Autodesk Fusion 360 part; units mm, degrees
note: some values were not read from the file. Chosen so that the rebuilt part matches the saved one: which face or edge a step refers to. Set by a fixed rule: which sketch regions a step uses.
(part 3 of 4)
sketch "Contents" plane through (0, 0, 0) normal (0, 0, 1) x (1, 0, 0) in component "Brace"
  circle A0 centre (34, 34.6) radius 15
  line L0 (40, 122) -> (22, 122)
  line L1 (60, 0) -> (0, 0) construction
  line L2 (18.5, 19.1) -> (18.5, 50.1) construction
  circle A1 centre (53, 31) radius 1.25
  circle A2 centre (53, 61) radius 1.25
  circle A3 centre (53, 121) radius 1.25
  line L3 (0, 0) -> (0, 182) construction
  line L4 (49.5, 19.1) -> (18.5, 50.1) construction
  circle A4 centre (18.5, 50.1) radius 1.5
  circle A5 centre (53, 91) radius 1.25
  line L5 (49.5, 50.1) -> (49.5, 19.1) construction
  line L6 (22, 162) -> (40, 162)
  line L7 (18.5, 19.1) -> (49.5, 50.1) construction
  circle A6 centre (53, 151) radius 1.25
  circle A7 centre (49.5, 19.1) radius 1.5
  line L8 (18.5, 50.1) -> (49.5, 50.1) construction
  line L9 (49.5, 19.1) -> (18.5, 19.1) construction
  line L10 (0, 182) -> (60, 182) construction
  circle A8 centre (18.5, 19.1) radius 1.5
  circle A9 centre (49.5, 50.1) radius 1.5
  line L11 (40, 162) -> (40, 122)
  line L12 (60, 182) -> (60, 0) construction
  line L13 (3.175, 95) -> (13.175, 95)
  line L14 (13.175, 95) -> (13.175, 87)
  line L15 (13.175, 87) -> (3.175, 87)
  line L16 (0, 425.6) -> (0, -184)
  line L17 (27.6442, 147.907) -> (28.3894, 146.7583)
  line L18 (34.519, 148.0232) -> (33.9924, 147.4295)
  arc A10 (33.9924, 147.4295) -> (27.6442, 147.907) centre (31, 150.0839) ccw
  line L19 (32, 141.3873) -> (32, 132.9489)
  line L20 (30, 132.9489) -> (30, 141.316)
  line L21 (31.1201, 154.0821) -> (30.7651, 146.624) construction
  line L22 (30, 132.9489) -> (32, 132.9489)
  arc A11 (34.519, 148.0232) -> (32, 141.3873) centre (42, 141.3873) ccw
  arc A12 (30, 141.316) -> (28.3894, 146.7583) centre (20, 141.316) ccw
  line L23 (31, 150.0839) -> (31, 109.1329) construction
  line L24 (19.1457, 161.9685) -> (15.5387, 161.9685)
  line L25 (15.5387, 161.9685) -> (15.5387, 153.7089)
  line L26 (19.1457, 161.1035) -> (22, 161.1035)
  line L27 (22, 158.4561) -> (22, 154.2014)
  line L28 (19.1457, 157.1289) -> (19.1457, 158.4561)
  line L29 (19.1457, 158.4561) -> (22, 158.4561)
  line L30 (22, 158.4561) -> (22, 157.1289)
  line L31 (19.1457, 153.7089) -> (19.1457, 158.4561)
  line L32 (19.1457, 161.1035) -> (19.1457, 161.9685)
  line L33 (15.5387, 153.7089) -> (19.1457, 153.7089)
  line L34 (22, 122) -> (22, 158.4561)
  line L35 (22, 161.1035) -> (22, 162)
  point P0 (60, 91)
  point P1 (34, 34.6)
  point P2 (0, 182)
  dimension "d1134" = 33
  dimension "d1135" = -30
  dimension "d1136" = 182
  dimension "d1137" = 60
  dimension "d974" = 2.5
  dimension "d975" = 7
  dimension "d1140" = 31
  dimension "d1141" = 31
  dimension "d1142" = 30
  dimension "d1143" = 3
  dimension "d1144" = 3
  dimension "d1145" = 3
  dimension "d1146" = 3
  dimension "d1147" = 26
  dimension "d1148" = 34.6
  dimension "d1149" = 20
  dimension "d1011" = 20
  dimension "d1012" = 18
  dimension "d1013" = 40
  dimension "d1716" = 3.175
  dimension "d1717" = 8
  dimension "d1718" = 87
  dimension "d1719" = 10
  dimension "d1720" = 9
  dimension "d1721" = 8
  dimension "d1722" = 2
  dimension "d1723" = 10
  dimension "d1724" = 10
  constraint perpendicular L1 L12
  constraint parallel L3 L12
  constraint coincident P2 L3.end
  constraint perpendicular L10 L12
  constraint midpoint P0 L12
  constraint horizontal P0 A5.centre
  constraint horizontal L9
  constraint perpendicular L2 L9
  constraint parallel L8 L9
  constraint parallel L2 L5
  constraint coincident P1 L4
  constraint coincident P1 L7
  constraint coincident P1 A0.centre
  constraint coincident L2.end L4.end
  constraint coincident L5.start L7.end
  constraint coincident L4.start L5.end
  constraint coincident L2.start L7.start
  constraint horizontal L6
  constraint vertical L11
  constraint horizontal L0
  constraint vertical L34
  constraint coincident L1.end L3.start
  constraint horizontal L13
  constraint vertical L14
  constraint horizontal L15
  constraint tangent L18 A10
  constraint tangent L17 A10
  constraint parallel L19 L20
  constraint coincident A10 L21.start
  constraint horizontal L22
  constraint tangent L18 A11
  constraint tangent L19 A11
  constraint tangent L17 A12
  constraint tangent L20 A12
  constraint coincident A10.centre L23.start
  constraint perpendicular L0 L23
  constraint horizontal L24
  constraint vertical L25
  constraint vertical L31
  constraint horizontal L26
  constraint vertical L27
  constraint coincident L27.end L34
  constraint coincident L26.start L31
  constraint vertical L28
  constraint horizontal L29
  constraint vertical L30
  constraint coincident L30.end L34
  constraint collinear L31 L32
  constraint perpendicular L31 L33
  constraint coincident L26.end L34
  constraint collinear L34 L35
  measures "d1136" distance of L1.end P2
  measures "d1137" distance of L1.end L1.start
  measures "d974" diameter of A5
  measures "d975" distance of A5.centre L12
  measures "d1140" distance of L2.end L5.start
  measures "d1141" distance of L2.end L2.start
  measures "d1142" diameter of A0
  measures "d1143" diameter of A4
  measures "d1144" diameter of A9
  measures "d1145" diameter of A7
  measures "d1146" diameter of A8
  measures "d1147" distance of P1 L12
  measures "d1148" distance of P1 L1
  measures "d1149" distance of L6.start L10
  measures "d1011" distance of L11 L12
  measures "d1012" distance of L0.end L0.start
  measures "d1013" distance of L0.end L6.start
  measures "d1716" distance of L13.start L16
  measures "d1717" distance of L13.end L14.end
  measures "d1718" distance of L10 L13
  measures "d1719" distance of L13.start L13.end
  measures "d1720" distance of A10.centre L34
  measures "d1721" diameter of A10
  measures "d1722" distance of L19.end L20.start
  measures "d1723" radius of A11
  measures "d1724" radius of A12
sketch "Content" plane through (0, 0, 0) normal (0, 0, 1) x (1, 0, 0) in component "Top"
  line L0 (-132, 172) -> (-116, 172)
  circle A0 centre (-49, 80) radius 1.5
  circle A1 centre (-49, 102) radius 1.5
  line L1 (0, 0) -> (-240, 0) construction
  line L2 (-114, 170) -> (-114, 127.9999)
  line L3 (-240, 182) -> (0, 182) construction
  line L4 (0, 182) -> (0, 0) construction
  circle A2 centre (-58, 151) radius 1.5
  circle A3 centre (-53, 136) radius 1.5
  circle A4 centre (-48, 151) radius 1.5
  circle A5 centre (-68, 146) radius 1.5
  circle A6 centre (-48, 146) radius 1.5
  circle A7 centre (-48, 156) radius 1.5
  circle A8 centre (-58, 156) radius 1.5
  circle A9 centre (-63, 141) radius 1.5
  circle A10 centre (-63, 151) radius 1.5
  circle A11 centre (-63, 146) radius 1.5
  circle A12 centre (-48, 141) radius 1.5
  circle A13 centre (-58, 146) radius 1.5
  circle A14 centre (-68, 151) radius 1.5
  line L5 (-163.976, 90) -> (-163.976, 96)
  circle A15 centre (-68, 136) radius 1.5
  circle A16 centre (-63, 156) radius 1.5
  circle A17 centre (-68, 156) radius 1.5
  circle A18 centre (-48, 136) radius 1.5
  circle A19 centre (-58, 136) radius 1.5
  line L6 (-240, 0) -> (-240, 182) construction
  circle A20 centre (-191, 102) radius 1.5
  circle A21 centre (-53, 156) radius 1.5
  circle A22 centre (-191, 80) radius 1.5
  line L7 (-134, 128) -> (-134, 170)
  circle A23 centre (-53, 146) radius 1.5
  line L8 (-159.976, 88) -> (-161.976, 88)
  line L9 (-161.976, 98) -> (-159.976, 98)
  circle A24 centre (-63, 136) radius 1.5
  line L10 (-157.976, 96) -> (-157.976, 90)
  circle A25 centre (-53, 141) radius 1.5
  circle A26 centre (-58, 141) radius 1.5
  circle A27 centre (-53, 151) radius 1.5
  line L11 (-116, 125.9999) -> (-132, 126)
  circle A28 centre (-68, 141) radius 1.5
  line L12 (0, 1.75) -> (0, 22.5)
  line L13 (1.75, 0) -> (22.5, 0)
  circle A29 centre (-68, 131) radius 1.5
  circle A30 centre (-63, 131) radius 1.5
  circle A31 centre (-58, 131) radius 1.5
  circle A32 centre (-53, 131) radius 1.5
  circle A33 centre (-48, 131) radius 1.5
  arc A34 (-161.976, 98) -> (-163.976, 96) centre (-161.976, 96) ccw
  arc A35 (-163.976, 90) -> (-161.976, 88) centre (-161.976, 90) ccw
  arc A36 (-159.976, 88) -> (-157.976, 90) centre (-159.976, 90) ccw
  arc A37 (-157.976, 96) -> (-159.976, 98) centre (-159.976, 96) ccw
  arc A38 (-132, 172) -> (-134, 170) centre (-132, 170) ccw
  arc A39 (-114, 170) -> (-116, 172) centre (-116, 170) ccw
  arc A40 (-116, 125.9999) -> (-114, 127.9999) centre (-116, 127.9999) ccw
  arc A41 (-134, 128) -> (-132, 126) centre (-132, 128) ccw
  line L14 (-131.3, 149.5) -> (-115.3, 149.5)
  circle A42 centre (-47, 47) radius 1.5
  circle A43 centre (-37, 62) radius 1.5
  circle A44 centre (-52, 47) radius 1.5
  circle A45 centre (-57, 67) radius 1.5
  circle A46 centre (-57, 57) radius 1.5
  circle A47 centre (-47, 67) radius 1.5
  circle A48 centre (-52, 57) radius 1.5
  circle A49 centre (-57, 47) radius 1.5
  circle A50 centre (-42, 62) radius 1.5
  circle A51 centre (-52, 52) radius 1.5
  circle A52 centre (-47, 62) radius 1.5
  circle A53 centre (-37, 52) radius 1.5
  circle A54 centre (-47, 52) radius 1.5
  circle A55 centre (-57, 62) radius 1.5
  circle A56 centre (-47, 57) radius 1.5
  circle A57 centre (-52, 67) radius 1.5
  circle A58 centre (-42, 52) radius 1.5
  circle A59 centre (-42, 57) radius 1.5
  circle A60 centre (-57, 52) radius 1.5
  circle A61 centre (-42, 47) radius 1.5
  circle A62 centre (-37, 67) radius 1.5
  circle A63 centre (-52, 62) radius 1.5
  circle A64 centre (-42, 67) radius 1.5
  circle A65 centre (-37, 57) radius 1.5
  circle A66 centre (-37, 47) radius 1.5
  line L15 (-242, 182) -> (-242, 0)
  circle A67 centre (-57, 42) radius 1.5
  circle A68 centre (-52, 42) radius 1.5
  circle A69 centre (-47, 42) radius 1.5
  circle A70 centre (-42, 42) radius 1.5
  circle A71 centre (-37, 42) radius 1.5
  circle A72 centre (-210, 15) radius 1.5
  circle A73 centre (-215, 30) radius 1.5
  circle A74 centre (-205, 25) radius 1.5
  circle A75 centre (-205, 30) radius 1.5
  circle A76 centre (-195, 20) radius 1.5
  circle A77 centre (-200, 30) radius 1.5
  circle A78 centre (-210, 20) radius 1.5
  circle A79 centre (-205, 15) radius 1.5
  circle A80 centre (-210, 30) radius 1.5
  circle A81 centre (-210, 10) radius 1.5
  circle A82 centre (-200, 10) radius 1.5
  circle A83 centre (-210, 25) radius 1.5
  circle A84 centre (-215, 25) radius 1.5
  circle A85 centre (-215, 15) radius 1.5
  circle A86 centre (-200, 25) radius 1.5
  circle A87 centre (-200, 20) radius 1.5
  circle A88 centre (-215, 10) radius 1.5
  circle A89 centre (-215, 20) radius 1.5
  circle A90 centre (-205, 10) radius 1.5
  circle A91 centre (-195, 10) radius 1.5
  circle A92 centre (-195, 25) radius 1.5
  circle A93 centre (-205, 20) radius 1.5
  circle A94 centre (-195, 15) radius 1.5
  circle A95 centre (-195, 30) radius 1.5
  circle A96 centre (-200, 15) radius 1.5
  line L16 (-240, 0) -> (-240, 182)
  circle A97 centre (-128.0762, 158.5418) radius 1.6
  circle A98 centre (-128.0762, 158.5418) radius 3.5
  circle A99 centre (-119.0762, 158.5418) radius 1.6
  circle A100 centre (-119.0762, 158.5418) radius 3.5
  circle A101 centre (-128.0762, 167.5418) radius 1.6
  circle A102 centre (-128.0762, 167.5418) radius 3.5
  circle A103 centre (-119.0762, 167.5418) radius 1.6
  circle A104 centre (-119.0762, 167.5418) radius 3.5
  arc A105 (-124.6, 139.8073) -> (-127.2667, 146.606) centre (-134.6, 139.8073) ccw
  line L17 (-124.6, 128.3707) -> (-122.8, 152.6283) construction
  arc A106 (-119.9333, 146.606) -> (-122.6, 139.8073) centre (-112.6, 139.8073) ccw
  line L18 (-124.6, 128.3707) -> (-124.6, 139.8073)
  line L19 (-122.6, 128.3707) -> (-124.6, 128.3707)
  line L20 (-122.6, 128.3707) -> (-124.6, 152.6283) construction
  line L21 (-122.6, 139.8073) -> (-122.6, 128.3707)
  arc A107 (-119.9333, 146.606) -> (-127.2667, 146.606) centre (-123.6, 150.0053) ccw
  point P0 (-134, 172)
  point P1 (-160.976, 126.0001)
  point P2 (-157.976, 98)
  point P3 (-114, 172)
  point P4 (-134, 126)
  point P5 (-160.976, 98)
  point P6 (-163.976, 98)
  point P7 (-163.976, 88)
  point P8 (-123.6526, 141.1379)
  dimension "d1161" = 142
  dimension "d1163" = 240
  dimension "d1164" = 182
  dimension "d1165" = 20
  dimension "d1166" = 46
  dimension "d1167" = 6
  dimension "d1168" = 10
  dimension "d1169" = 10
  dimension "d1170" = 106
  dimension "d1171" = 84
  dimension "d1172" = 26
  dimension "d1173" = 3
  dimension "d1174" = 68
  dimension "d1175" = 3
  dimension "d1176" = 49
  dimension "d1177" = 80
  dimension "d1600" = 2
  dimension "d1601" = 2
  dimension "d1602" = 2
  dimension "d1603" = 2
  dimension "d1604" = 2
  dimension "d1605" = 2
  dimension "d1606" = 2
  dimension "d1607" = 2
  dimension "d1696" = 3
  dimension "d1699" = 47
  dimension "d1700" = 47
  dimension "d1705" = 3
  dimension "d1707" = 30
  dimension "d1708" = 20
  dimension "d1709" = 3.2
  dimension "d1710" = 7
  dimension "d1713" = 9
  dimension "d1714" = 9
  dimension "d1739" = 1.8
  dimension "d1740" = 10
  dimension "d1741" = 10
  dimension "d1742" = 10
  constraint horizontal L3
  constraint perpendicular L3 L4
  constraint horizontal L0
  constraint vertical L2
  constraint vertical L7
  constraint horizontal L9
  constraint vertical L10
  constraint horizontal L8
  constraint vertical L5
  constraint vertical P1 P5
  constraint perpendicular L1 L6
  constraint collinear L4 L12
  constraint collinear L1 L13
  constraint coincident P5 L9
  constraint coincident P6 L9
  constraint coincident P6 L5
  constraint tangent L9 A34
  constraint tangent L5 A34
  constraint coincident P7 L8
  constraint coincident P7 L5
  constraint tangent L8 A35
  constraint tangent L5 A35
  constraint tangent L8 A36
  constraint tangent L10 A36
  constraint coincident P2 L10
  constraint coincident P2 L9
  constraint tangent L10 A37
  constraint tangent L9 A37
  constraint coincident P0 L0
  constraint coincident P0 L7
  constraint tangent L0 A38
  constraint tangent L7 A38
  constraint coincident P3 L0
  constraint coincident P3 L2
  constraint tangent L0 A39
  constraint tangent L2 A39
  constraint coincident P1 L11
  constraint tangent L11 A40
  constraint tangent L2 A40
  constraint coincident P4 L7
  constraint coincident P4 L11
  constraint tangent L7 A41
  constraint tangent L11 A41
  constraint equal L0 L11
  constraint midpoint P5 L9
  constraint concentric A97 A98
  constraint horizontal L19
  constraint perpendicular L18 L19
  constraint parallel L18 L21
  constraint coincident P8 L20
  constraint coincident P8 L17
  constraint tangent A106 A107
  constraint tangent A106 L21
  constraint tangent A105 A107
  constraint tangent A105 L18
  measures "d1163" distance of L3.end L3.start
  measures "d1164" distance of L1.end L3.start
  measures "d1165" distance of P0 P3
  measures "d1166" distance of P0 P4
  measures "d1167" distance of P2 P6
  measures "d1168" distance of P6 P7
  measures "d1169" distance of L0 L3
  measures "d1170" distance of L6 L7
  measures "d1171" distance of L3 L9
  measures "d1172" distance of A17.centre L3
  measures "d1173" diameter of A17
  measures "d1174" distance of A17.centre L4
  measures "d1175" diameter of A20
  measures "d1176" distance of A20.centre L6
  measures "d1177" distance of A20.centre L3
  measures "d1600" radius of A34
  measures "d1601" radius of A35
  measures "d1602" radius of A36
  measures "d1603" radius of A37
  measures "d1604" radius of A38
  measures "d1605" radius of A39
  measures "d1606" radius of A40
  measures "d1607" radius of A41
  measures "d1696" diameter of A45
  measures "d1699" distance of L4 A47.centre
  measures "d1700" distance of L1 A49.centre
  measures "d1705" diameter of A73
  measures "d1707" distance of A80.centre L16
  measures "d1708" distance of L1 A93.centre
  measures "d1709" diameter of A97
  measures "d1710" diameter of A98
  measures "d1739" distance of L20.end L17.end
  measures "d1740" diameter of A107
  measures "d1741" radius of A106
  measures "d1742" radius of A105
sketch "Content (2)" plane through (0, 0, 0) normal (0, 0, 1) x (1, 0, 0) in component "Bottom"
  line L0 (-240, -184) -> (-240, -2) construction
  line L1 (-240, -2) -> (0, -2) construction
  line L2 (0, -184) -> (-240, -184) construction
  circle A0 centre (-139, -9) radius 1
  circle A1 centre (-15, -172) radius 1.75
  line L3 (0, -2) -> (0, -184) construction
  circle A2 centre (-120, -93.901) radius 1.05
  circle A3 centre (-225, -172) radius 1.75
  circle A4 centre (-225, -17) radius 1.75
  circle A5 centre (-139, -103) radius 1
  circle A6 centre (-15, -17) radius 1.75
  circle A7 centre (-233, -103) radius 1
  circle A8 centre (-233, -9) radius 1
  line L4 (1.75, 0) -> (22.5, 0) construction
  line L5 (0, 1.75) -> (0, 22.5) construction
  line L6 (0, -184) -> (-304.8, -184)
  circle A9 centre (-76.675, -120) radius 2
  circle A10 centre (-26.675, -120) radius 2
  circle A11 centre (-76.675, -151) radius 2
  circle A12 centre (-26.675, -151) radius 2
  line L7 (0, 425.6) -> (0, -184)
  circle A13 centre (-211.0542, -25.3538) radius 1.0005
  circle A14 centre (-157.9209, -25.3538) radius 1.0005
  circle A15 centre (-104.7876, -25.3538) radius 1.0005
  circle A16 centre (-51.6542, -25.3538) radius 1.0005
  circle A17 centre (-211.0542, -68.4205) radius 1.0005
  circle A18 centre (-157.9209, -68.4205) radius 1.0005
  circle A19 centre (-51.6542, -68.4205) radius 1.0005
  circle A20 centre (-211.0542, -111.4871) radius 1.0005
  circle A21 centre (-51.6542, -111.4871) radius 1.0005
  circle A22 centre (-211.0542, -154.5538) radius 1.0005
  circle A23 centre (-157.9209, -154.5538) radius 1.0005
  circle A24 centre (-104.7876, -154.5538) radius 1.0005
  circle A25 centre (-51.6542, -154.5538) radius 1.0005
  point P0 (-120, -93.901)
  point P1 (0, -2)
  dimension "d828" = 210
  dimension "d829" = -155
  dimension "d832" = 94
  dimension "d833" = -94
  dimension "d282" = 3.5
  dimension "d289" = 2
  dimension "d422" = 240
  dimension "d423" = 182
  dimension "d424" = 15
  dimension "d426" = 15
  dimension "d427" = 7
  dimension "d428" = 7
  dimension "d463" = 2.1
  dimension "d843" = 2
  dimension "d1634" = 4
  dimension "d1637" = 50
  dimension "d1638" = -31
  dimension "d1639" = 64
  dimension "d1640" = 26.675
  dimension "d1726" = 2.001
  dimension "d1729" = 159.4
  dimension "d1730" = -129.2
  constraint horizontal L2
  constraint perpendicular L0 L2
  constraint parallel L1 L2
  constraint coincident P0 A2.centre
  constraint coincident P1 L1.end
  constraint vertical L3
  constraint collinear L3 L5
  measures "d282" diameter of A4
  measures "d289" diameter of A8
  measures "d422" distance of P1 L0.end
  measures "d423" distance of L0.start L0.end
  measures "d424" distance of A4.centre L1
  measures "d426" distance of A4.centre L0
  measures "d427" distance of A8.centre L1
  measures "d428" distance of A8.centre L0
  measures "d463" diameter of A2
  measures "d843" distance of L1 L4
  measures "d1634" diameter of A9
  measures "d1639" distance of L2 A9.centre
  measures "d1640" distance of A12.centre L7
  measures "d1726" diameter of A13
sketch "Content (3)" plane through (0, 0, 0) normal (0, 0, 1) x (1, 0, 0) in component "Front"
  line L0 (242, 62) -> (2, 62) construction
  line L1 (2, 2) -> (242, 2) construction
  line L2 (2, 62) -> (2, 2) construction
  line L3 (242, 62) -> (242, 2) construction
  line L4 (0, 1.75) -> (0, 22.5) construction
  line L5 (1.75, 0) -> (22.5, 0) construction
  line L6 (39.175, 22.1755) -> (39.175, 46.6727) construction
  circle A0 centre (48.175, 16.175) radius 5
  circle A1 centre (48.175, 34.175) radius 9
  circle A2 centre (216.325, 32) radius 15
  circle A3 centre (216.325, 32) radius 1.5
  circle A4 centre (216.325, 56.5) radius 1.5
  circle A5 centre (216.325, 7.5) radius 1.5
  circle A6 centre (216.325, 32) radius 20.5 construction
  circle A7 centre (169.325, 32) radius 20.5 construction
  circle A8 centre (169.325, 32) radius 15
  circle A9 centre (169.325, 7.5) radius 1.5
  circle A10 centre (169.325, 32) radius 1.5
  circle A11 centre (169.325, 56.5) radius 1.5
  circle A12 centre (122.325, 32) radius 20.5 construction
  circle A13 centre (122.325, 32) radius 15
  circle A14 centre (122.325, 7.5) radius 1.5
  circle A15 centre (122.325, 32) radius 1.5
  circle A16 centre (122.325, 56.5) radius 1.5
  point P0 (1.401, 31.401)
  point P1 (47.095, 2)
  point P2 (242, 32)
  dimension "d492" = 240
  dimension "d493" = 60
  dimension "d1106" = 2
  dimension "d1400" = 2
  dimension "d1567" = 14.175
  dimension "d1568" = 10
  dimension "d1569" = 18
  dimension "d1570" = 18
  dimension "d1725" = 46.175
  dimension "d1746" = 30
  dimension "d1748" = 3
  dimension "d1751" = 0
  dimension "d1752" = -24.5
  dimension "d1753" = 41
  dimension "d1754" = 25.675
  dimension "d1757" = -47
  dimension "d1758" = 0
  constraint perpendicular L0 L2
  constraint perpendicular L0 L3
  constraint horizontal L1
  constraint vertical L6
  constraint vertical A0.centre A1.centre
  constraint tangent L6 A1
  constraint midpoint L3 P2
  constraint horizontal A2.centre P2
  constraint concentric A2 A3
  constraint concentric A2 A6
  measures "d492" distance of L0.end L0.start
  measures "d493" distance of L1.end L0.start
  measures "d1106" distance of L2 L4
  measures "d1400" distance of L1 L5
  measures "d1567" distance of L1 A0.centre
  measures "d1568" diameter of A0
  measures "d1569" diameter of A1
  measures "d1570" vertical distance of A0.centre A1.centre
  measures "d1725" distance of L2 A1.centre
  measures "d1746" diameter of A2
  measures "d1748" diameter of A3
  measures "d1753" diameter of A6
  measures "d1754" distance of L3 A2.centre
sketch "Content (4)" plane through (0, 0, 0) normal (0, 0, 1) x (1, 0, 0) in component "Back"
  line L0 (128, -33) -> (128, -39)
  line L1 (116, -39) -> (116, -33)
  circle A0 centre (172, -18) radius 1.75
  circle A1 centre (182, -28) radius 1.75
  circle A2 centre (182, -18) radius 1.75
  line L2 (2, -6) -> (2, -66) construction
  line L3 (119, -30) -> (125, -30)
  line L4 (242, -6) -> (2, -6) construction
  line L5 (2, -66) -> (242, -66) construction
  circle A3 centre (56, -27) radius 1.5
  circle A4 centre (172, -28) radius 1.75
  circle A5 centre (71, -17) radius 1.5
  circle A6 centre (56, -17) radius 1.5
  circle A7 centre (46, -32) radius 1.5
  circle A8 centre (223.2, -48) radius 5.5
  line L6 (242, -66) -> (242, -6) construction
  circle A9 centre (66, -32) radius 1.5
  circle A10 centre (66, -22) radius 1.5
  circle A11 centre (61, -32) radius 1.5
  circle A12 centre (41, -27) radius 1.5
  circle A13 centre (71, -32) radius 1.5
  circle A14 centre (46, -17) radius 1.5
  circle A15 centre (56, -22) radius 1.5
  circle A16 centre (66, -17) radius 1.5
  circle A17 centre (56, -32) radius 1.5
  circle A18 centre (66, -27) radius 1.5
  circle A19 centre (61, -22) radius 1.5
  circle A20 centre (61, -17) radius 1.5
  circle A21 centre (46, -22) radius 1.5
  circle A22 centre (51, -22) radius 1.5
  line L7 (125, -42) -> (119, -42)
  circle A23 centre (41, -32) radius 1.5
  circle A24 centre (51, -32) radius 1.5
  circle A25 centre (41, -17) radius 1.5
  circle A26 centre (71, -27) radius 1.5
  circle A27 centre (46, -27) radius 1.5
  circle A28 centre (51, -27) radius 1.5
  circle A29 centre (61, -27) radius 1.5
  circle A30 centre (51, -17) radius 1.5
  circle A31 centre (41, -22) radius 1.5
  circle A32 centre (71, -22) radius 1.5
  line L8 (0, 1.75) -> (0, 22.5) construction
  line L9 (1.75, 0) -> (22.5, 0) construction
  circle A33 centre (192, -18) radius 1.75
  circle A34 centre (202, -18) radius 1.75
  circle A35 centre (192, -28) radius 1.75
  circle A36 centre (202, -28) radius 1.75
  line L10 (14.1495, -52.3784) -> (48.441, -52.3784) construction
  line L11 (48.441, -52.3784) -> (48.441, -46.5889) construction
  line L12 (48.441, -46.5889) -> (14.1495, -46.5889) construction
  line L13 (14.1495, -46.5889) -> (14.1495, -52.3784) construction
  arc A37 (119, -30) -> (116, -33) centre (119, -33) ccw
  arc A38 (128, -33) -> (125, -30) centre (125, -33) ccw
  arc A39 (125, -42) -> (128, -39) centre (125, -39) ccw
  arc A40 (116, -39) -> (119, -42) centre (119, -39) ccw
  line L14 (227, -16) -> (227, -26)
  line L15 (220.6, -14) -> (225, -14)
  line L16 (225, -28) -> (220.6, -28)
  line L17 (218.6, -26) -> (218.6, -16)
  arc A41 (220.6, -14) -> (218.6, -16) centre (220.6, -16) ccw
  arc A42 (227, -16) -> (225, -14) centre (225, -16) ccw
  arc A43 (218.6, -26) -> (220.6, -28) centre (220.6, -26) ccw
  arc A44 (225, -28) -> (227, -26) centre (225, -26) ccw
  point P0 (242, -36)
  point P1 (116, -42)
  point P2 (116, -30)
  point P3 (128, -30)
  point P4 (218.6, -28)
  point P5 (218.6, -14)
  point P6 (227, -14)
  point P7 (223.2, -28)
  dimension "d1005" = 5
  dimension "d1006" = 5
  dimension "d1009" = 10
  dimension "d1010" = -10
  dimension "d502" = 240
  dimension "d503" = 60
  dimension "d696" = 18
  dimension "d866" = 12
  dimension "d867" = 12
  dimension "d869" = 24
  dimension "d870" = 3
  dimension "d1039" = 34
  dimension "d1041" = 12
  dimension "d1179" = 18.8
  dimension "d1180" = 114
  dimension "d1183" = 39
  dimension "d1047" = 2
  dimension "d1048" = 6
  dimension "d1561" = 3.5
  dimension "d1562" = 11
  dimension "d1563" = 70
  dimension "d1596" = 3
  dimension "d1597" = 3
  dimension "d1598" = 3
  dimension "d1599" = 3
  dimension "d1646" = 8.4
  dimension "d1647" = 14
  dimension "d1648" = 8
  dimension "d1654" = 2
  dimension "d1655" = 2
  dimension "d1656" = 2
  dimension "d1657" = 2
  dimension "d1658" = 15
  constraint horizontal L5
  constraint vertical L6
  constraint vertical L2
  constraint midpoint P0 L6
  constraint horizontal L4
  constraint horizontal L3
  constraint vertical L0
  constraint horizontal L7
  constraint vertical L1
  constraint coincident P2 L1
  constraint coincident P2 L3
  constraint tangent L1 A37
  constraint tangent L3 A37
  constraint coincident P3 L3
  constraint coincident P3 L0
  constraint tangent L3 A38
  constraint tangent L0 A38
  constraint tangent L0 A39
  constraint tangent L7 A39
  constraint coincident P1 L1
  constraint coincident P1 L7
  constraint tangent L1 A40
  constraint tangent L7 A40
  constraint horizontal L15
  constraint vertical L14
  constraint horizontal L16
  constraint vertical L17
  constraint vertical A8.centre P7
  constraint coincident P5 L17
  constraint coincident P5 L15
  constraint tangent L17 A41
  constraint tangent L15 A41
  constraint coincident P6 L15
  constraint coincident P6 L14
  constraint tangent L15 A42
  constraint tangent L14 A42
  constraint coincident L16 P7
  constraint coincident P4 L17
  constraint coincident P4 L16
  constraint tangent L17 A43
  constraint tangent L16 A43
  constraint tangent L14 A44
  constraint tangent L16 A44
  measures "d502" distance of L5.end L2.end
  measures "d503" distance of L2.end L2.start
  measures "d696" distance of A8.centre L5
  measures "d866" distance of P2 P3
  measures "d867" distance of P1 P2
  measures "d869" distance of L5 L7
  measures "d870" diameter of A23
  measures "d1039" distance of A23.centre L5
  measures "d1041" distance of A0.centre L4
  measures "d1179" distance of A8.centre L6
  measures "d1180" distance of L0 L6
  measures "d1183" distance of A23.centre L2
  measures "d1047" distance of L2 L8
  measures "d1048" distance of L4 L9
  measures "d1561" diameter of A0
  measures "d1562" diameter of A8
  measures "d1563" distance of A0.centre L6
  measures "d1596" radius of A37
  measures "d1597" radius of A38
  measures "d1598" radius of A39
  measures "d1599" radius of A40
  measures "d1646" distance of P5 P6
  measures "d1647" distance of P4 P5
  measures "d1648" distance of L4 L15
  measures "d1654" radius of A41
  measures "d1655" radius of A42
  measures "d1656" radius of A43
  measures "d1657" radius of A44
  measures "d1658" distance of L6 L14
sketch "Content (5)" plane through (0, 0, 0) normal (0, 0, 1) x (1, 0, 0) in component "Right"
  line L0 (-302, 182) -> (-242, 182) construction
  circle A0 centre (-275, 112) radius 5.75
  circle A1 centre (-277, 80) radius 1.75
  circle A2 centre (-287, 100) radius 1.75
  circle A3 centre (-277, 90) radius 1.75
  line L1 (-264.7, 57.5) -> (-267, 57.5)
  line L2 (-267, 45) -> (-264.7, 45)
  circle A4 centre (-287, 90) radius 1.75
  circle A5 centre (-287, 80) radius 1.75
  line L3 (-269, 55.5) -> (-269, 47)
  line L4 (-262.7, 47) -> (-262.7, 55.5)
  circle A6 centre (-297, 151) radius 1
  circle A7 centre (-277, 100) radius 1.75
  circle A8 centre (-297, 61) radius 1
  circle A9 centre (-297, 121) radius 1
  circle A10 centre (-297, 91) radius 1
  line L5 (-242, 182) -> (-242, 0) construction
  circle A11 centre (-297, 31) radius 1
  line L6 (-302, 0) -> (-302, 182) construction
  circle A12 centre (-267, 80) radius 1.75
  line L7 (-242, 0) -> (-302, 0) construction
  circle A13 centre (-267, 90) radius 1.75
  circle A14 centre (-267, 100) radius 1.75
  line L8 (1.75, 0) -> (22.5, 0) construction
  line L9 (0, 1.75) -> (0, 22.5) construction
  arc A15 (-262.7, 55.5) -> (-264.7, 57.5) centre (-264.7, 55.5) ccw
  arc A16 (-267, 57.5) -> (-269, 55.5) centre (-267, 55.5) ccw
  arc A17 (-269, 47) -> (-267, 45) centre (-267, 47) ccw
  arc A18 (-264.7, 45) -> (-262.7, 47) centre (-264.7, 47) ccw
  point P0 (-242, 91)
  point P1 (-262.7, 45)
  point P2 (-272, 0)
  point P3 (-269, 45)
  point P4 (-269, 57.5)
  point P5 (-302, 182)
  point P6 (-272, 182)
  dimension "d960" = -10
  dimension "d961" = -10
  dimension "d964" = 0
  dimension "d965" = -30
  dimension "d846" = 2
  dimension "d910" = 182
  dimension "d911" = 60
  dimension "d923" = 11.5
  dimension "d924" = 70
  dimension "d925" = 27
  dimension "d927" = 33
  dimension "d929" = 6.3
  dimension "d930" = 3.5
  dimension "d1192" = 100
  dimension "d1194" = 91
  dimension "d992" = 12.5
  dimension "d993" = 242
  dimension "d1538" = 45
  dimension "d1540" = 15
  dimension "d1564" = 5
  dimension "d1642" = 2
  dimension "d1643" = 2
  dimension "d1644" = 2
  dimension "d1645" = 2
  constraint perpendicular L5 L7
  constraint parallel L5 L6
  constraint coincident P5 L0.start
  constraint perpendicular L0 L5
  constraint midpoint P2 L7
  constraint midpoint P6 L0
  constraint horizontal L2
  constraint horizontal L1
  constraint vertical L3
  constraint midpoint P0 L5
  constraint perpendicular L1 L4
  constraint collinear L7 L8
  constraint tangent L1 A15
  constraint tangent L4 A15
  constraint coincident P4 L1
  constraint coincident P4 L3
  constraint tangent L1 A16
  constraint tangent L3 A16
  constraint coincident P3 L3
  constraint coincident P3 L2
  constraint tangent L3 A17
  constraint tangent L2 A17
  constraint coincident P1 L2
  constraint coincident P1 L4
  constraint tangent L2 A18
  constraint tangent L4 A18
  measures "d846" diameter of A10
  measures "d910" distance of L6.start P5
  measures "d911" distance of L6.start L5.end
  measures "d923" diameter of A0
  measures "d924" distance of A0.centre L0
  measures "d925" distance of A0.centre L6
  measures "d927" distance of L3 L6
  measures "d929" distance of P1 P3
  measures "d930" diameter of A14
  measures "d1192" distance of A14.centre L7
  measures "d1194" distance of A10.centre L7
  measures "d992" distance of P3 P4
  measures "d993" distance of L5 L9
  measures "d1538" distance of L2 L7
  measures "d1540" distance of A2.centre L6
  measures "d1564" distance of A10.centre L6
  measures "d1642" radius of A15
  measures "d1643" radius of A16
  measures "d1644" radius of A17
  measures "d1645" radius of A18
sketch "Content (6)" plane through (0, 0, 0) normal (0, 0, 1) x (1, 0, 0) in component "Left"
  circle A0 centre (-246.401, -121.7005) radius 1
  line L0 (-242, 0) -> (-242, -183.401)
  line L1 (-302, -183.401) -> (-302, -1.401)
  circle A1 centre (-246.401, -31.7005) radius 1
  circle A2 centre (-246.401, -151.7005) radius 1
  circle A3 centre (-246.401, -61.7005) radius 1
  circle A4 centre (-247, -91.7005) radius 1
  line L2 (0, 1.75) -> (0, 22.5) construction
  line L3 (-302, -1.401) -> (-242, -1.401)
  line L4 (-242, -183.401) -> (-302, -183.401)
  line L5 (1.75, 0) -> (22.5, 0) construction
  line L6 (-242, 0) -> (-302, 0)
  circle A5 centre (-247.5, -159.401) radius 1.5
  circle A6 centre (-272, -159.401) radius 20.5 construction
  circle A7 centre (-272, -159.401) radius 15
  circle A8 centre (-296.5, -159.401) radius 1.5
  line L7 (-296.5, -159.401) -> (-247.5, -159.401) construction
  circle A9 centre (-272, -113.401) radius 20.5 construction
  circle A10 centre (-296.5, -113.401) radius 1.5
  line L8 (-296.5, -113.401) -> (-247.5, -113.401) construction
  circle A11 centre (-272, -113.401) radius 15
  circle A12 centre (-272, -67.401) radius 20.5 construction
  circle A13 centre (-296.5, -67.401) radius 1.5
  line L9 (-296.5, -67.401) -> (-247.5, -67.401) construction
  circle A14 centre (-272, -67.401) radius 15
  circle A15 centre (-247.5, -113.401) radius 1.5
  circle A16 centre (-247.5, -67.401) radius 1.5
  circle A17 centre (-262.9095, -67.5364) radius 3.5
  circle A18 centre (-262.9095, -67.5364) radius 1.6
  circle A19 centre (-267.3375, -59.5961) radius 1.6
  circle A20 centre (-267.3375, -59.5961) radius 3.5
  circle A21 centre (-276.428, -59.4607) radius 1.6
  circle A22 centre (-276.428, -59.4607) radius 3.5
  circle A23 centre (-281.0905, -67.2656) radius 1.6
  circle A24 centre (-281.0905, -67.2656) radius 3.5
  circle A25 centre (-276.6625, -75.2059) radius 1.6
  circle A26 centre (-276.6625, -75.2059) radius 3.5
  circle A27 centre (-267.572, -75.3413) radius 1.6
  circle A28 centre (-267.572, -75.3413) radius 3.5
  arc A29 (-267.7994, -108.87) -> (-270.4355, -115.6711) centre (-260.4356, -115.6357) ccw
  line L10 (-270.4355, -115.6711) -> (-270.3981, -126.2293)
  line L11 (-272.3981, -126.2293) -> (-272.4354, -115.699)
  line L12 (-270.3981, -126.2293) -> (-272.4073, -102.4695) construction
  arc A30 (-267.7994, -108.87) -> (-275.1326, -108.9029) centre (-271.4813, -105.4871) ccw
  arc A31 (-272.4354, -115.699) -> (-275.1326, -108.9029) centre (-282.4354, -115.7344) ccw
  line L13 (-272.3981, -126.2293) -> (-270.6073, -102.4695) construction
  line L14 (-272.3981, -126.2293) -> (-270.3981, -126.2293)
  arc A32 (-267.7994, -155.07) -> (-275.1326, -155.1029) centre (-271.4813, -151.6871) ccw
  arc A33 (-267.7994, -155.07) -> (-270.4355, -161.8711) centre (-260.4356, -161.8357) ccw
  line L15 (-272.3981, -172.4293) -> (-272.4354, -161.899)
  line L16 (-270.4355, -161.8711) -> (-270.3981, -172.4293)
  line L17 (-295.901, -159.601) -> (-246.901, -159.601) construction
  arc A34 (-272.4354, -161.899) -> (-275.1326, -155.1029) centre (-282.4354, -161.9344) ccw
  line L18 (-272.3981, -172.4293) -> (-270.6073, -148.6695) construction
  line L19 (-270.3981, -172.4293) -> (-272.4073, -148.6695) construction
  line L20 (-272.3981, -172.4293) -> (-270.3981, -172.4293)
  point P0 (-241.401, -91.7005)
  point P1 (-301.401, -92.401)
  point P2 (-302, -1.401)
  point P3 (-278.401, 0)
  point P4 (-272, -183.401)
  point P5 (-271.4556, -113.7241)
  point P6 (-271.4556, -159.9241)
  point P7 (-271.401, -159.601)
  point P8 (-271.401, -159.601)
  dimension "d523" = 182
  dimension "d861" = 5
  dimension "d1401" = 242
  dimension "d1542" = 60
  dimension "d1763" = 30
  dimension "d1765" = 41
  dimension "d1766" = 3
  dimension "d1767" = 24.5
  dimension "d1768" = 24.5
  dimension "d1769" = 24
  dimension "d1772" = 0
  dimension "d1773" = 46
  dimension "d1778" = 3.2
  dimension "d1779" = 7
  dimension "d1783" = 360
  dimension "d1788" = 1.8
  dimension "d1789" = 10
  dimension "d1790" = 10
  dimension "d1791" = 10
  dimension "d1792" = 1.8
  dimension "d1793" = 10
  dimension "d1794" = 10
  dimension "d1795" = 10
  constraint parallel L0 L1
  constraint coincident P2 L1.end
  constraint horizontal L4
  constraint coincident L1.start L4.end
  constraint coincident L0.start L6.start
  constraint concentric A6 A7
  constraint coincident A8.centre L7.start
  constraint coincident A5.centre L7.end
  constraint coincident A6.centre L7
  constraint equal A5 A8
  constraint horizontal L7
  constraint midpoint L4 P4
  constraint vertical A6.centre P4
  constraint concentric A17 A18
  constraint parallel L10 L11
  constraint coincident P5 L12
  constraint coincident P5 L13
  constraint tangent A29 A30
  constraint tangent A29 L10
  constraint tangent A30 A31
  constraint tangent L11 A31
  constraint horizontal L14
  constraint parallel L15 L16
  constraint coincident P6 L19
  constraint coincident P6 L18
  constraint tangent A32 A33
  constraint tangent A33 L16
  constraint tangent A32 A34
  constraint tangent L15 A34
  constraint horizontal L20
  measures "d523" distance of P2 L1.start
  measures "d861" distance of A4.centre L0
  measures "d1401" distance of L0 L2
  measures "d1542" distance of L0.end L1.start
  measures "d1763" diameter of A7
  measures "d1765" diameter of A6
  measures "d1766" diameter of A5
  measures "d1767" distance of A8.centre A6.centre
  measures "d1768" distance of A5.centre A6.centre
  measures "d1769" distance of L4 A6.centre
  measures "d1778" diameter of A18
  measures "d1779" diameter of A17
  measures "d1788" distance of L12.end L13.end
  measures "d1789" diameter of A30
  measures "d1790" radius of A29
  measures "d1791" radius of A31
  measures "d1792" distance of L19.end L18.end
  measures "d1793" diameter of A32
  measures "d1794" radius of A33
  measures "d1795" radius of A34
sketch "Teeth" plane through (0, 0, 0) normal (0, 0, 1) x (1, 0, 0) in component "Front"
  line L0 (86, 6.3042) -> (86, 15.7758)
  line L1 (89.175, 6.3042) -> (89.175, 15.7758)
  line L2 (87.6137, 36.905) -> (87.5613, 36.905)
  line L3 (87.5613, 27.095) -> (87.6137, 27.095)
  line L4 (87.6137, 16.905) -> (87.5613, 16.905)
  line L5 (89.175, 35.7758) -> (89.175, 28.2242)
  line L6 (89.175, 48.2242) -> (89.175, 57.6958)
  line L7 (86, 57.6958) -> (86, 48.2242)
  line L8 (242, 62) -> (242, 2) construction
  line L9 (2, 2) -> (242, 2) construction
  line L10 (2, 62) -> (2, 2) construction
  arc A0 (87.6137, 16.905) -> (86, 15.7758) centre (86.7071, 16.4829) ccw
  arc A1 (89.175, 15.7758) -> (87.5613, 16.905) centre (88.4679, 16.4829) ccw
  arc A2 (87.5613, 27.095) -> (89.175, 28.2242) centre (88.4679, 27.5171) ccw
  arc A3 (86, 28.2242) -> (87.6137, 27.095) centre (86.7071, 27.5171) ccw
  line L11 (86, 28.2242) -> (86, 35.7758)
  arc A4 (89.175, 35.7758) -> (87.5613, 36.905) centre (88.4679, 36.4829) ccw
  arc A5 (87.6137, 36.905) -> (86, 35.7758) centre (86.7071, 36.4829) ccw
  arc A6 (87.5613, 47.095) -> (89.175, 48.2242) centre (88.4679, 47.5171) ccw
  arc A7 (86, 48.2242) -> (87.6137, 47.095) centre (86.7071, 47.5171) ccw
  line L12 (0, 1.75) -> (0, 22.5) construction
  line L13 (87.5613, 47.095) -> (87.6137, 47.095)
  line L14 (87.6137, 58.825) -> (87.5613, 58.825)
  line L15 (2, 62) -> (242, 62) construction
  line L16 (1.75, 0) -> (22.5, 0)
  line L17 (87.6137, 5.175) -> (87.5613, 5.175)
  arc A8 (87.6137, 58.825) -> (86, 57.6958) centre (86.7071, 58.4029) ccw
  arc A9 (89.175, 57.6958) -> (87.5613, 58.825) centre (88.4679, 58.4029) ccw
  arc A10 (86, 6.3042) -> (87.6137, 5.175) centre (86.7071, 5.5971) ccw
  arc A11 (87.5613, 5.175) -> (89.175, 6.3042) centre (88.4679, 5.5971) ccw
  dimension "d1086" = 2
  dimension "d1087" = 0.4221
  dimension "d1091" = 10.19
  dimension "d1094" = 2
  dimension "d1109" = 0.4221
  dimension "d1113" = 2
  dimension "d1116" = 3.175
  dimension "d1117" = 0.7071
  dimension "d1221" = 2
  dimension "d1222" = 2
  dimension "d1223" = 2
  dimension "d1224" = 2
  dimension "d1225" = 2
  dimension "d1227" = 0.7071
  dimension "d1228" = 0.7071
  dimension "d1229" = 0.4221
  dimension "d1230" = 0.4221
  dimension "d1232" = 0.4221
  dimension "d1233" = 0.4221
  dimension "d1235" = 0.7071
  dimension "d1236" = 0.7071
  dimension "d1178" = 0.7071
  dimension "d1323" = 240
  dimension "d1324" = 84
  dimension "d1399" = 2
  dimension "d1454" = 3.175
  dimension "d1456" = 0.4221
  dimension "d1457" = 0.4221
  dimension "d1460" = 60
  dimension "d1461" = 2
  dimension "d1462" = 3.175
  dimension "d1463" = 3.175
  dimension "d1466" = 9.81
  dimension "d1468" = 14.905
  dimension "d1469" = 14.905
  dimension "d1471" = 10.19
  dimension "d1472" = 0.7071
  dimension "d1473" = 0.7071
  dimension "d1571" = 2
  dimension "d1573" = 2
  dimension "d1574" = 0.7071
  dimension "d1575" = 0.7071
  dimension "d1576" = 0.4221
  dimension "d1577" = 0.4221
  dimension "d1578" = 2
  dimension "d1579" = 2
  dimension "d1580" = 0.4221
  dimension "d1581" = 0.4221
  dimension "d1582" = 0.7071
  dimension "d1583" = 0.7071
  constraint vertical L7
  constraint vertical L6
  constraint horizontal L3
  constraint horizontal L2
  constraint vertical L5
  constraint collinear L1 L5
  constraint perpendicular L9 L10
  constraint collinear L0 L11
  constraint collinear L7 L11
  constraint horizontal L13
  constraint perpendicular L7 L14
  constraint perpendicular L8 L15
  constraint perpendicular L0 L17
  measures "d1086" diameter of A0
  measures "d1087" distance of A0.centre L4
  measures "d1091" distance of L3 L4
  measures "d1094" diameter of A7
  measures "d1109" distance of A5.centre L2
  measures "d1113" diameter of A5
  measures "d1116" distance of L6 L7
  measures "d1117" distance of A7.centre L7
  measures "d1221" diameter of A1
  measures "d1222" diameter of A2
  measures "d1223" diameter of A4
  measures "d1224" diameter of A3
  measures "d1225" diameter of A6
  measures "d1227" distance of A6.centre L6
  measures "d1228" distance of A0.centre L0
  measures "d1229" distance of A1.centre L4
  measures "d1230" distance of A2.centre L3
  measures "d1232" distance of A3.centre L3
  measures "d1233" distance of A4.centre L2
  measures "d1235" distance of A4.centre L5
  measures "d1236" distance of A2.centre L5
  measures "d1178" distance of A1.centre L1
  measures "d1323" distance of L10.start L8.start
  measures "d1324" distance of L0 L10
  measures "d1399" distance of L10 L12
  measures "d1454" distance of L5 L11
  measures "d1456" distance of A6.centre L13
  measures "d1457" distance of A7.centre L13
  measures "d1460" distance of L9 L15
  measures "d1461" distance of L9 L16
  measures "d1462" distance of L14 L15
  measures "d1463" distance of L9 L17
  measures "d1466" distance of L2 L3
  measures "d1468" distance of L4 L9
  measures "d1469" distance of L13 L15
  measures "d1471" distance of L2 L13
  measures "d1472" distance of A3.centre L11
  measures "d1473" distance of A5.centre L11
  measures "d1571" diameter of A10
  measures "d1573" diameter of A11
  measures "d1574" distance of L0 A10.centre
  measures "d1575" distance of L1 A11.centre
  measures "d1576" distance of L17 A11.centre
  measures "d1577" distance of L17 A10.centre
  measures "d1578" diameter of A8
  measures "d1579" diameter of A9
  measures "d1580" distance of L14 A8.centre
  measures "d1581" distance of L14 A9.centre
  measures "d1582" distance of L7 A8.centre
  measures "d1583" distance of L6 A9.centre
sketch "Teeth (2)" plane through (0, 0, 0) normal (0, 0, 1) x (1, 0, 0) in component "Back"
  arc A0 (86, -39.7758) -> (87.6137, -40.905) centre (86.7071, -40.4829) ccw
  arc A1 (89.175, -52.2242) -> (87.5613, -51.095) centre (88.4679, -51.5171) ccw
  line L0 (2, -6) -> (2, -66) construction
  line L1 (87.6137, -31.095) -> (87.5613, -31.095)
  line L2 (89.175, -32.2242) -> (89.175, -39.7758)
  line L3 (89.175, -61.6958) -> (89.175, -52.2242)
  line L4 (87.5613, -20.905) -> (87.6137, -20.905)
  line L5 (86, -10.3042) -> (86, -19.7758)
  arc A2 (89.175, -32.2242) -> (87.5613, -31.095) centre (88.4679, -31.5171) ccw
  arc A3 (87.6137, -31.095) -> (86, -32.2242) centre (86.7071, -31.5171) ccw
  arc A4 (87.5613, -20.905) -> (89.175, -19.7758) centre (88.4679, -20.4829) ccw
  arc A5 (86, -19.7758) -> (87.6137, -20.905) centre (86.7071, -20.4829) ccw
  line L6 (87.5613, -40.905) -> (87.6137, -40.905)
  line L7 (89.175, -19.7758) -> (89.175, -10.3042)
  line L8 (86, -61.6958) -> (86, -52.2242)
  line L9 (87.6137, -51.095) -> (87.5613, -51.095)
  arc A6 (87.6137, -51.095) -> (86, -52.2242) centre (86.7071, -51.5171) ccw
  arc A7 (87.5613, -40.905) -> (89.175, -39.7758) centre (88.4679, -40.4829) ccw
  line L10 (2, -6) -> (80.576, -6) construction
  line L11 (242, -6) -> (242, -66) construction
  line L12 (0, 1.75) -> (0, 22.5) construction
  line L13 (1.75, 0) -> (22.5, 0) construction
  line L14 (86, -32.2242) -> (86, -39.7758)
  line L15 (77.401, -66) -> (242, -66) construction
  line L16 (2, -66) -> (77.401, -66) construction
  line L17 (87.6137, -62.825) -> (87.5613, -62.825)
  line L18 (80.576, -6) -> (242, -6) construction
  line L19 (87.6137, -9.175) -> (87.5613, -9.175)
  arc A8 (87.5613, -62.825) -> (89.175, -61.6958) centre (88.4679, -62.4029) ccw
  arc A9 (86, -61.6958) -> (87.6137, -62.825) centre (86.7071, -62.4029) ccw
  arc A10 (87.6137, -9.175) -> (86, -10.3042) centre (86.7071, -9.5971) ccw
  arc A11 (89.175, -10.3042) -> (87.5613, -9.175) centre (88.4679, -9.5971) ccw
  dimension "d1404" = 2
  dimension "d1405" = 0.4221
  dimension "d1406" = 10.19
  dimension "d1407" = 2
  dimension "d1408" = 0.4221
  dimension "d1409" = 2
  dimension "d1412" = 0.7071
  dimension "d1413" = 2
  dimension "d1414" = 2
  dimension "d1415" = 2
  dimension "d1416" = 2
  dimension "d1417" = 2
  dimension "d1418" = 0.7071
  dimension "d1419" = 0.7071
  dimension "d1420" = 0.4221
  dimension "d1421" = 0.4221
  dimension "d1423" = 0.4221
  dimension "d1424" = 0.4221
  dimension "d1425" = 0.7071
  dimension "d1426" = 0.7071
  dimension "d1427" = 0.7071
  dimension "d1428" = 240
  dimension "d1429" = 84
  dimension "d1431" = 14.905
  dimension "d1433" = 9.81
  dimension "d1436" = 2
  dimension "d1437" = 14.905
  dimension "d1440" = 6
  dimension "d1441" = 0.4221
  dimension "d1442" = 0.4221
  dimension "d1443" = 0.7071
  dimension "d1444" = 0.7071
  dimension "d1446" = 3.175
  dimension "d1447" = 3.175
  dimension "d1451" = 3.175
  dimension "d1452" = 60
  dimension "d1453" = 3.175
  dimension "d1470" = 10.19
  dimension "d1584" = 2
  dimension "d1585" = 2
  dimension "d1586" = 0.7071
  dimension "d1587" = 0.4221
  dimension "d1588" = 0.4221
  dimension "d1589" = 0.7071
  dimension "d1590" = 2
  dimension "d1591" = 2
  dimension "d1592" = 0.7071
  dimension "d1593" = 0.7071
  dimension "d1594" = 0.4221
  dimension "d1595" = 0.4221
  constraint vertical L5
  constraint vertical L7
  constraint horizontal L6
  constraint horizontal L1
  constraint vertical L2
  constraint collinear L2 L3
  constraint perpendicular L0 L10
  constraint perpendicular L0 L16
  constraint collinear L8 L14
  constraint perpendicular L8 L17
  constraint collinear L5 L14
  constraint perpendicular L5 L19
  measures "d1404" diameter of A6
  measures "d1405" distance of A6.centre L9
  measures "d1406" distance of L6 L9
  measures "d1407" diameter of A5
  measures "d1408" distance of A3.centre L1
  measures "d1409" diameter of A3
  measures "d1412" distance of A5.centre L5
  measures "d1413" diameter of A1
  measures "d1414" diameter of A7
  measures "d1415" diameter of A2
  measures "d1416" diameter of A0
  measures "d1417" diameter of A4
  measures "d1418" distance of A4.centre L7
  measures "d1419" distance of A6.centre L8
  measures "d1420" distance of A1.centre L9
  measures "d1421" distance of A7.centre L6
  measures "d1423" distance of A0.centre L6
  measures "d1424" distance of A2.centre L1
  measures "d1425" distance of A2.centre L2
  measures "d1426" distance of A7.centre L2
  measures "d1427" distance of A1.centre L3
  measures "d1428" distance of L0.start L11.start
  measures "d1429" distance of L0 L8
  measures "d1431" distance of L9 L15
  measures "d1433" distance of L1 L6
  measures "d1436" distance of L0 L12
  measures "d1437" distance of L4 L10
  measures "d1440" distance of L10 L13
  measures "d1441" distance of A5.centre L4
  measures "d1442" distance of A4.centre L4
  measures "d1443" horizontal distance of A3.centre A3.end
  measures "d1444" distance of A0.centre L14
  measures "d1446" distance of L5 L7
  measures "d1447" distance of L2 L14
  measures "d1451" distance of L16 L17
  measures "d1452" distance of L10 L15
  measures "d1453" distance of L10 L19
  measures "d1470" distance of L1 L4
  measures "d1584" diameter of A9
  measures "d1585" diameter of A8
  measures "d1586" distance of L8 A9.centre
  measures "d1587" distance of L17 A9.centre
  measures "d1588" distance of L17 A8.centre
  measures "d1589" distance of L3 A8.centre
  measures "d1590" diameter of A10
  measures "d1591" diameter of A11
  measures "d1592" distance of L5 A10.centre
  measures "d1593" distance of L7 A11.centre
  measures "d1594" distance of L19 A10.centre
  measures "d1595" distance of L19 A11.centre